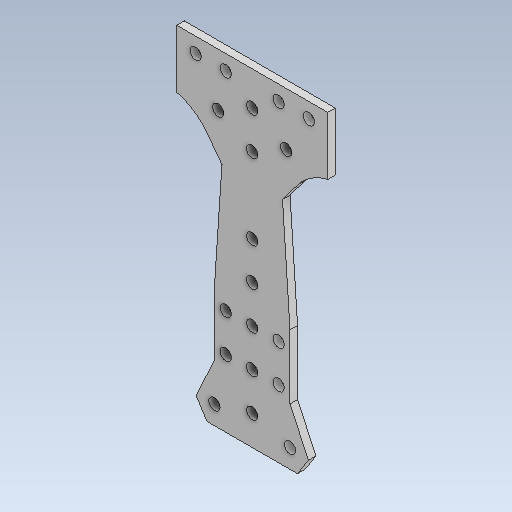
# Autodesk Inventor part: body_bone_3
Saved by Autodesk Inventor 2020 (Build 240168000, 168)
## iProperties
Created: 2019-05-16
Part Number: body_bone_3
Material: Generic
Document SubType Name: Modeling
Designer: psrob
Density: 1 g/cm^3
Appearance: Default
Author: psrob
Autodesk Inventor part; units mm, degrees
ref_plane "YZ Plane" through (0, 0, 0) normal (1, 0, 0) x (0, 1, 0)
ref_plane "XZ Plane" through (0, 0, 0) normal (0, 1, 0) x (-1, 0, 0)
ref_plane "XY Plane" through (0, 0, 0) normal (0, 0, 1) x (1, 0, 0)
sketch "Sketch1" plane through (0, 0, 0) normal (0, 0, 1) x (1, 0, 0)
  circle A0 centre (-34, 4) radius 1.5
  circle A1 centre (-30, 13) radius 1.5
  circle A2 centre (-27, 4) radius 1.5
  line L0 (-30, 23) -> (-30, 40)
  line L1 (-39.076923, 9.384615) -> (-30, 23)
  line L2 (-40, 0) -> (-40, 8)
  line L3 (-40, 0) -> (-20, 0)
  line L4 (-20, 0) -> (-20, 40)
  line L5 (-20, 40) -> (-30, 40)
  circle A3 centre (-6, 4) radius 1.5
  circle A4 centre (-10, 13) radius 1.5
  circle A5 centre (-13, 4) radius 1.5
  line L6 (-10, 23) -> (-10, 40)
  line L7 (-20, 40) -> (-10, 40)
  line L8 (-20, 0) -> (-20, 40)
  line L9 (0, 0) -> (-20, 0)
  line L10 (0, 0) -> (0, 8)
  line L11 (-0.923077, 9.384615) -> (-10, 23)
  line L12 (-3, 8) -> (-37, 8)
  circle A6 centre (-29, 80.883435) radius 1.5
  circle A7 centre (-27, 90.883435) radius 1.5
  circle A8 centre (-35, 90.883435) radius 1.5
  line L13 (-40, 79.500979) -> (-40, 94.883435)
  arc A9 (-32.05, 74.283435) -> (-40, 79.500979) centre (-43.25, 65.883435) ccw
  line L14 (-28.021661, 68.912316) -> (-32.05, 74.283435)
  line L15 (-20, 68.912316) -> (-28.021661, 68.912316)
  line L16 (-20, 94.883435) -> (-20, 68.912316)
  line L17 (-40, 94.883435) -> (-20, 94.883435)
  circle A10 centre (-11, 80.883435) radius 1.5
  circle A11 centre (-13, 90.883435) radius 1.5
  circle A12 centre (-5, 90.883435) radius 1.5
  line L18 (0, 79.500979) -> (0, 94.883435)
  line L19 (0, 94.883435) -> (-20, 94.883435)
  line L20 (-20, 94.883435) -> (-20, 68.912316)
  line L21 (-20, 68.912316) -> (-11.978339, 68.912316)
  line L22 (-11.978339, 68.912316) -> (-7.95, 74.283435)
  arc A13 (0, 79.500979) -> (-7.95, 74.283435) centre (3.25, 65.883435) ccw
  line L23 (-10, 40) -> (-11.978339, 68.912316)
  line L24 (-28.021661, 68.912316) -> (-30, 40)
  constraints: 4 end point
sketch "Sketch1 outline for Extrusion1" plane through (0, 0, 0) normal (0, 0, 1) x (1, 0, 0)
  line L0 (-37, 8) -> (-3, 8)
  line L1 (-30, 23) -> (-37, 8)
  line L2 (-3, 8) -> (-10, 23)
  line L3 (-30, 40) -> (-30, 23)
  line L4 (-10, 23) -> (-10, 40)
  line L5 (-28.021661, 68.912316) -> (-30, 40)
  line L6 (-10, 40) -> (-11.978339, 68.912316)
  line L7 (-32.05, 74.283435) -> (-28.021661, 68.912316)
  line L8 (-11.978339, 68.912316) -> (-7.95, 74.283435)
  arc A0 (-40, 79.500979) -> (-32.05, 74.283435) centre (-43.25, 65.883435) cw
  arc A1 (-7.95, 74.283435) -> (0, 79.500979) centre (3.25, 65.883435) cw
  line L9 (-40, 94.883435) -> (-40, 79.500979)
  line L10 (0, 79.500979) -> (0, 94.883435)
  line L11 (-20, 94.883435) -> (-40, 94.883435)
  line L12 (0, 94.883435) -> (-20, 94.883435)
  circle A2 centre (-30, 13) radius 1.5
  circle A3 centre (-10, 13) radius 1.5
  circle A4 centre (-29, 80.883435) radius 1.5
  circle A5 centre (-35, 90.883435) radius 1.5
  circle A6 centre (-27, 90.883435) radius 1.5
  circle A7 centre (-13, 90.883435) radius 1.5
  circle A8 centre (-11, 80.883435) radius 1.5
  circle A9 centre (-5, 90.883435) radius 1.5
extrude "Extrusion1" add sketch "Sketch1 outline for Extrusion1" along normal blind 2
chamfer "Chamfer1" distance 5 angle 45 2 edges at (-37, 8, 1) (-3, 8, 1)
sketch "Sketch2" plane through (0, 0, 2) normal (0, 0, 1) x (1, 0, 0)
  circle A0 centre (-27, 35.883435) radius 1.5
  circle A1 centre (-13, 35.883435) radius 1.5
  circle A2 centre (-13, 25.883435) radius 1.5
  circle A3 centre (-27, 25.883435) radius 1.5
  circle A4 centre (-20, 75.883435) radius 1.5
  circle A5 centre (-20, 25.883435) radius 1.5
  circle A6 centre (-20, 15.883435) radius 1.5
  circle A7 centre (-20, 35.883435) radius 1.5
  circle A8 centre (-20, 85.883435) radius 1.5
  line L0 (-5, 8) -> (-2.773501, 12.160251)
  line L1 (-5, 8) -> (-35, 8)
  line L2 (-37.226499, 12.160251) -> (-35, 8)
  line L3 (-37.226499, 12.160251) -> (-30, 23)
  line L4 (-30, 23) -> (-30, 40)
  line L5 (-30, 40) -> (-26, 40)
  arc A9 (-26, 40) -> (-23, 43) centre (-26, 43) ccw
  line L6 (-23, 43) -> (-23, 65.912316)
  arc A10 (-23, 65.912316) -> (-26, 68.912316) centre (-26, 65.912316) ccw
  line L7 (-26, 68.912316) -> (-28.021661, 68.912316)
  line L8 (-28.021661, 68.912316) -> (-32.05, 74.283435)
  arc A11 (-32.05, 74.283435) -> (-40, 79.500979) centre (-43.25, 65.883435) ccw
  line L9 (-40, 79.500979) -> (-40, 94.883435)
  line L10 (-40, 94.883435) -> (0, 94.883435)
  line L11 (0, 94.883435) -> (0, 79.500979)
  arc A12 (0, 79.500979) -> (-7.95, 74.283435) centre (3.25, 65.883435) ccw
  line L12 (-7.95, 74.283435) -> (-11.978339, 68.912316)
  line L13 (-11.978339, 68.912316) -> (-14, 68.912316)
  arc A13 (-14, 68.912316) -> (-17, 65.912316) centre (-14, 65.912316) ccw
  line L14 (-17, 65.912316) -> (-17, 43)
  arc A14 (-17, 43) -> (-14, 40) centre (-14, 43) ccw
  line L15 (-14, 40) -> (-10, 40)
  line L16 (-10, 40) -> (-10, 23)
  line L17 (-10, 23) -> (-2.773501, 12.160251)
  circle A15 centre (-30, 13) radius 1.5
  circle A16 centre (-27, 90.883435) radius 1.5
  circle A17 centre (-29, 80.883435) radius 1.5
  circle A18 centre (-35, 90.883435) radius 1.5
  circle A19 centre (-11, 80.883435) radius 1.5
  circle A20 centre (-13, 90.883435) radius 1.5
  circle A21 centre (-5, 90.883435) radius 1.5
  circle A22 centre (-10, 13) radius 1.5
  point P0 (0, 0)
extrude "Extrusion2" cut sketch "Sketch2" against normal blind 10 contours A0 | A1 | A2 | A3 | A4 | A5 | A6 | A7 | A8
sketch "Sketch3" plane through (0, 0, 2) normal (0, 0, 1) x (1, 0, 0)
  circle A0 centre (-13, 35.883435) radius 1.5
  circle A1 centre (-20, 35.883435) radius 1.5
  circle A2 centre (-27, 35.883435) radius 1.5
  circle A3 centre (-13, 25.883435) radius 1.5
  circle A4 centre (-20, 75.883435) radius 1.5
  circle A5 centre (-20, 25.883435) radius 1.5
  circle A6 centre (-27, 25.883435) radius 1.5
  circle A7 centre (-20, 15.883435) radius 1.5
  circle A8 centre (-20, 85.883435) radius 1.5
  line L0 (-5.114427, 12.530916) -> (-8, 8)
  line L1 (-5.114427, 12.530916) -> (-10, 23)
  line L2 (-10, 23) -> (-10, 40)
  line L3 (-10, 40) -> (-11.978339, 68.912316)
  line L4 (-11.978339, 68.912316) -> (-7.95, 74.283435)
  arc A9 (0, 79.500979) -> (-7.95, 74.283435) centre (3.25, 65.883435) ccw
  line L5 (0, 79.500979) -> (0, 94.883435)
  line L6 (0, 94.883435) -> (-40, 94.883435)
  line L7 (-40, 94.883435) -> (-40, 79.500979)
  arc A10 (-32.05, 74.283435) -> (-40, 79.500979) centre (-43.25, 65.883435) ccw
  line L8 (-32.05, 74.283435) -> (-28.021661, 68.912316)
  line L9 (-28.021661, 68.912316) -> (-30, 40)
  line L10 (-30, 40) -> (-30, 23)
  line L11 (-30, 23) -> (-34.885573, 12.530916)
  line L12 (-32, 8) -> (-34.885573, 12.530916)
  line L13 (-32, 8) -> (-8, 8)
  circle A11 centre (-13, 90.883435) radius 1.5
  circle A12 centre (-11, 80.883435) radius 1.5
  circle A13 centre (-5, 90.883435) radius 1.5
  circle A14 centre (-29, 80.883435) radius 1.5
  circle A15 centre (-27, 90.883435) radius 1.5
  circle A16 centre (-35, 90.883435) radius 1.5
  circle A17 centre (-30, 13) radius 1.5
  circle A18 centre (-10, 13) radius 1.5
  circle A19 centre (-20, 75.883435) radius 1.5
  line L14 (-20, 75.883435) -> (-20, 55.883435)
  line L15 (-20, 55.883435) -> (-20, 45.883435)
  circle A20 centre (-20, 55.883435) radius 1.5
  circle A21 centre (-20, 45.883435) radius 1.5
  point P0 (0, 0)
  dimension "d7" = 20
  dimension "d8" = 10
  dimension "d9" = 3
  dimension "d10" = 3
  constraints: 4 end point, 2 centre point, 2 coincident, 1 point on line, 1 vertical
  measures "d7" distance of L14.start L14.end
  measures "d8" distance of L14.end L15.end
  measures "d9" diameter of A20
  measures "d10" diameter of A21
extrude "Extrusion3" cut sketch "Sketch3" against normal blind 10 contours A20 L15 L14 | L14 L15 A20 | A21
body "Solid1"
